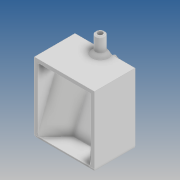
# Autodesk Inventor part: WaterDrainWell
Saved by Autodesk Inventor 2020 (Build 240168000, 168)
## iProperties
Created: 2019-08-07
Part Number: WaterDrainWell
Material: 일반
Document SubType Name: Modeling
Designer: Jeong Ji Hoon
Density: 1 g/cm^3
Appearance: 기본값
Author: Jeong Ji Hoon
## iProperties of the stored document _3D 인쇄.ipt
Created: 2019-08-07
Part Number: _3D 인쇄
Material: 일반
Document SubType Name: Modeling
Designer: Jeong Ji Hoon
Density: 1 g/cm^3
Appearance: 기본값
Author: Jeong Ji Hoon
Autodesk Inventor part; units mm, degrees
ref_plane "YZ Plane" through (0, 0, 0) normal (1, 0, 0) x (0, 1, 0)
ref_plane "XZ Plane" through (0, 0, 0) normal (0, 1, 0) x (-1, 0, 0)
ref_plane "XY Plane" through (0, 0, 0) normal (0, 0, 1) x (1, 0, 0)
sketch "스케치1" plane through (0, 0, 0) normal (0, 0, 1) x (1, 0, 0)
  line L0 (0, 0) -> (17, 0)
  line L1 (17, 0) -> (17, 20)
  line L2 (17, 20) -> (0, 20)
  line L3 (0, 20) -> (0, 0)
  dimension "d0" = 17
  dimension "d1" = 20
  constraints: 8 end point, 2 parallel, 1 horizontal, 1 perpendicular
  measures "d0" distance of L0.start L0.end
  measures "d1" distance of L0.end L1.end
extrude "돌출1" add sketch "스케치1" along normal blind 1.5
sketch "스케치2" plane through (0, 0, 1.5) normal (0, 0, 1) x (1, 0, 0)
  line L0 (0, 20) -> (0, 0) projected
  line L1 (0, 0) -> (17, 0) projected
  line L2 (17, 0) -> (17, 20) projected
  line L3 (17, 20) -> (0, 20) projected
  line L4 (1, 19) -> (1, 1)
  line L5 (1, 1) -> (16, 1)
  line L6 (16, 1) -> (16, 19)
  line L7 (16, 19) -> (1, 19)
  dimension "d4" = 1
  constraints: 8 end point, 3 other
  measures "d4" distance between parallel lines of L3 L7
extrude "돌출2" add sketch "스케치2" along normal blind 10
sketch "스케치3" plane through (1, 1, 1.5) normal (1, 0, 0) x (0, 0, -1)
  line L0 (0, 18) -> (0, 0) projected
  line L1 (0, 18) -> (-10, 18) projected
  line L2 (-10, 0) -> (-10, 18) projected
  line L3 (0, 0) -> (-10, 0) projected
  line L4 (-5, 0) -> (0, 13)
  line L5 (0, 16) -> (-8, 18)
  point P0 (1.5, -1)
  dimension "d7" = 13
  dimension "d8" = 5
  dimension "d9" = 2
  dimension "d10" = 2
  constraints: 4 end point, 3 point on line, 1 midpoint
  measures "d7" distance from line of L3 L4.end
  measures "d8" distance from line of L2 L4.start
  measures "d9" distance from line of L2 L5.end
  measures "d10" distance of L5.start L0.start
extrude "돌출3" add sketch "스케치3" along normal up to surface (15 mm away) contours L0 L5 L1 | L0 L3 L4
fillet "모깎기1" radius 1 3 edges at (0, 0, 5.75) (8.5, 0, 11.5) (17, 0, 5.75)
chamfer "모따기1" distance 5 distance2 5 1 edges at (1, 7.5, 4) measured on face at (1, 7.6795, 4.4667)
chamfer "모따기2" distance 5 distance2 5 1 edges at (16, 7.5, 4) measured on face at (16, 7.6795, 4.4667)
chamfer "모따기3" distance 2 angle 45 2 edges at (5.4615, 15.5, 1.5) (11.5385, 15.5, 1.5)
sketch "스케치4" plane through (1, 19, 9.5) normal (0, -0.9701425, 0.2425356) x (1, 0, 0)
  line L0 (8.952, -8.2462) -> (6.048, -8.2462) projected
  circle A0 centre (7.5, -7.6462) radius 0.7
  point P0 (-1, -13.8245)
  point P1 (7.5, -8.2462)
  point P2 (7.8606, -8.2462)
  point P3 (7.1394, -8.2462)
  dimension "d23" = 1.4
  dimension "d24" = 0.6
  constraints: 1 centre point, 1 midpoint, 1 vertical alignment
  measures "d23" diameter of A0
  measures "d24" distance of point (7.5, -8.246) A0.centre
extrude "돌출4" cut sketch "스케치4" against normal blind 10 contours L0 A0 picked at (7.5847, -7.817)
sketch "스케치5" plane through (0, 20, 0) normal (0, 1, 0) x (1, 0, 0)
  ellipse E0 centre (8.5, -1.3685) end of major axis (8.5, -0.6469) minor radius 0.7 (8.1394, -0.75) -> (8.8606, -0.75) ccw projected
  circle A0 centre (8.5, -1.3685) radius 1.3
  circle A1 centre (8.5, -1.3685) radius 0.7159
  point P0 (8.1394, -1.9869)
  point P1 (8.8606, -1.9869)
  point P2 (8.5, -2.6685)
  point P3 (7.2197, -1.5942)
  point P4 (8.8606, -0.75)
  dimension "d27" = 2.6
  dimension "d30" = 0.5841
  constraints: 2 coincident, 2 point on circle, 1 centre point, 4 other
  measures "d27" diameter of A0
extrude "돌출5" add sketch "스케치5" along normal blind 5 contours E0 A1 | A1 E0 | A0 picked at (7.7946, -1.337) picked at (9.2023, -1.3759)
chamfer "모따기4" distance 1 angle 45 1 edges at (7.2, 20, 1.3685)
sketch "스케치6" plane through (0, 0, 0) normal (0, 0, -1) x (-1, 0, 0)
  line L0 (-1, 0) -> (-16, 0) projected
  line L1 (-8.5, 7.5) -> (-6.3349, 6.25)
  line L2 (-6.3349, 6.25) -> (-6.3349, 3.75)
  line L3 (-6.3349, 3.75) -> (-8.5, 2.5)
  line L4 (-8.5, 2.5) -> (-10.6651, 3.75)
  line L5 (-10.6651, 3.75) -> (-10.6651, 6.25)
  line L6 (-10.6651, 6.25) -> (-8.5, 7.5)
  line L7 (-8.5, 17.5) -> (-6.3349, 16.25)
  line L8 (-6.3349, 16.25) -> (-6.3349, 13.75)
  line L9 (-6.3349, 13.75) -> (-8.5, 12.5)
  line L10 (-8.5, 12.5) -> (-10.6651, 13.75)
  line L11 (-10.6651, 13.75) -> (-10.6651, 16.25)
  line L12 (-10.6651, 16.25) -> (-8.5, 17.5)
  point P0 (0, 0)
  point P1 (-8.5, 5)
  point P2 (-8.5, 0)
  point P3 (-8.5, 15)
  point P4 (-8.5, 0)
  dimension "d36" = 5
  dimension "d37" = 5
  dimension "d38" = 5
  dimension "d39" = 10
  constraints: 24 end point, 4 vertical alignment, 2 midpoint, 26 other
  measures "d36" distance from line of L0 point (-8.5, 5)
  measures "d37" distance of L1.start L3.end
  measures "d38" distance of L12.end L9.end
  measures "d39" distance of point (-8.5, 5) point (-8.5, 15)
extrude "돌출6" add sketch "스케치6" along normal blind 3
chamfer "모따기5" distance 0.3 angle 45 1 edges at (7.2, 25, 1.3685)
fillet "모깎기3" radius 1 1 edges at (8.5, 17.3153, 2.7612)
